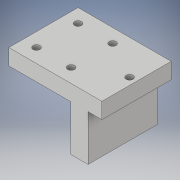
# Autodesk Inventor part: Vertical sedder motor spacer
Saved by Autodesk Inventor 2017 (Build 210142000, 142)
## iProperties
Created: 2017-05-24
Part Number: Vertical sedder motor spacer
Material: Generic
Document SubType Name: Modeling
Designer: Jon
Density: 1 g/cm^3
Appearance: Default
Author: Jon
Autodesk Inventor part; units mm, degrees
ref_plane "YZ Plane" through (0, 0, 0) normal (1, 0, 0) x (0, 1, 0)
ref_plane "XZ Plane" through (0, 0, 0) normal (0, 1, 0) x (-1, 0, 0)
ref_plane "XY Plane" through (0, 0, 0) normal (0, 0, 1) x (1, 0, 0)
sketch "Sketch1" plane through (0, 0, 0) normal (0, 1, 0) x (-1, 0, 0)
  line L0 (34.3343, 23.8125) -> (-51.0732, 23.8125)
  line L1 (-51.0732, 23.8125) -> (-51.0732, -39.6875)
  line L2 (-51.0732, -39.6875) -> (34.3343, -39.6875)
  line L3 (34.3343, -39.6875) -> (34.3343, 23.8125)
  point P0 (0, 0)
  dimension "d0" = 63.5
  dimension "d1" = 85.4075
  constraints: 8 end point, 2 parallel, 1 horizontal, 1 perpendicular
  measures "d0" distance of L2.end L0.start
  measures "d1" distance of L1.end L2.end
extrude "Extrusion1" add sketch "Sketch1" along normal blind 14.605
sketch "Sketch2" plane through (0, 0, 0) normal (0, -1, 0) x (1, 0, 0)
  line L0 (-34.3343, 23.8125) -> (51.0732, 23.8125) projected
  line L1 (32.0232, -39.6875) -> (38.3732, -39.6875)
  line L2 (38.3732, -39.6875) -> (38.3732, 23.8125)
  line L3 (38.3732, 23.8125) -> (32.0232, 23.8125)
  line L4 (32.0232, 13.0175) -> (32.0232, -28.8925)
  line L5 (51.0732, 23.8125) -> (51.0732, -39.6875) projected
  line L6 (22.4982, -39.6875) -> (38.3732, -39.6875)
  line L7 (38.3732, -39.6875) -> (38.3732, -28.8925)
  line L8 (32.0232, -28.8925) -> (22.4982, -28.8925)
  line L9 (22.4982, -28.8925) -> (22.4982, -39.6875)
  line L10 (22.4982, 23.8125) -> (38.3732, 23.8125)
  line L11 (38.3732, 23.8125) -> (38.3732, 13.0175)
  line L12 (32.0232, 13.0175) -> (22.4982, 13.0175)
  line L13 (22.4982, 13.0175) -> (22.4982, 23.8125)
  point P0 (0, 0)
  dimension "d4" = 63.5
  dimension "d5" = 6.35
  dimension "d6" = 12.7
  dimension "d15" = 10.795
  dimension "d16" = 10.795
  dimension "d17" = 15.875
  dimension "d18" = 15.875
  constraints: 24 end point, 6 parallel, 4 point on line, 3 horizontal, 3 perpendicular
  measures "d4" distance of L3.end L1.start
  measures "d5" distance of L1.start L1.end
  measures "d6" distance between parallel lines of L5 L2
  measures "d15" distance between parallel lines of L6 L8
  measures "d16" distance between parallel lines of L12 L10
  measures "d17" distance between parallel lines of L2 L13
  measures "d18" distance between parallel lines of L7 L9
extrude "Extrusion3" add sketch "Sketch2" along normal blind 41.91
sketch "Sketch4" plane through (0, 0, 0) normal (0, -1, 0) x (1, 0, 0)
  line L0 (22.4982, -39.6875) -> (-34.3343, -39.6875) projected
  line L1 (-34.3343, -39.6875) -> (-34.3343, 23.8125) projected
  line L2 (-34.3343, 23.8125) -> (22.4982, 23.8125) projected
  point P0 (0, 0)
  point P1 (-21.6343, -26.9875)
  point P2 (-21.6343, 11.1125)
  point P3 (10.1157, 11.1125)
  point P4 (10.1157, -26.9875)
  dimension "d21" = 12.7
  dimension "d22" = 12.7
  dimension "d23" = 12.7
  dimension "d24" = 12.7
  dimension "d25" = 12.7
  dimension "d26" = 12.7
  dimension "d27" = 44.45
  dimension "d28" = 44.45
  measures "d21" distance from line of L0 point (-21.634, -26.987)
  measures "d22" distance from line of point (-21.634, -26.987) L1
  measures "d23" distance from line of L1 point (-21.634, 11.112)
  measures "d24" distance from line of point (-21.634, 11.112) L2
  measures "d25" distance from line of L2 point (10.116, 11.112)
  measures "d26" distance from line of L0 point (10.116, -26.987)
  measures "d27" distance from line of L1 point (10.116, -26.987)
  measures "d28" distance from line of L1 point (10.116, 11.112)
hole "Hole1" at (-21.6343, 0, -26.9875) at (-21.6343, 0, 11.1125) at (10.1157, 0, 11.1125) at (10.1157, 0, -26.9875) direction (0, 1, 0) diameter 6.35 end through all
sketch "Sketch5" plane through (0, 0, 0) normal (0, -1, 0) x (1, 0, 0)
  line L0 (38.3732, -39.6875) -> (38.3732, 23.8125) projected
  line L1 (51.0732, 23.8125) -> (51.0732, -39.6875) projected
  line L2 (38.3732, 23.8125) -> (51.0732, 23.8125) projected
  point P0 (0, 0)
  point P1 (44.7232, -7.9375)
  dimension "d36" = 6.35
  dimension "d38" = 31.75
  measures "d36" distance from line of L0 point (44.723, -7.937)
  measures "d38" distance from line of L2 point (44.723, -7.937)
hole "Hole2" at (44.7232, 0, -7.9375) direction (0, 1, 0) diameter 6.35 end through all
equation "\"d23\" = d22"
equation "\"d24\" = d21"
equation "\"d25\" = d21"
equation "\"d26\" = d21"
equation "\"d28\" = d27"
body "Solid1"
